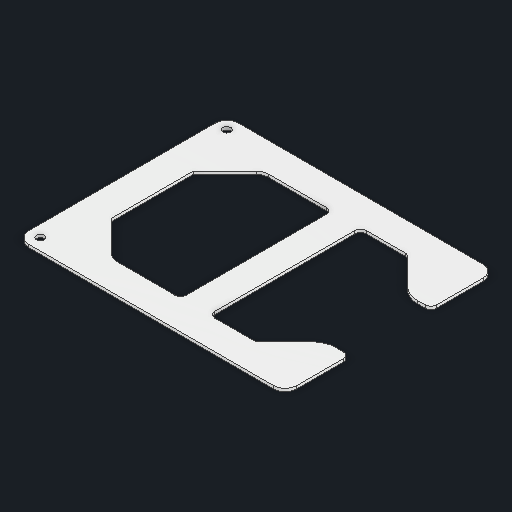
# Autodesk Inventor part: Compression Pads
Saved by Autodesk Inventor 2025.1 (Build 291241000, 241)
## iProperties
Created: 2024-11-12
Part Number: Compression Pads
Material: Acetal Resin, White
Document SubType Name: Sheet Metal
Designer: avere
Density: 1.425 g/cm^3
Appearance: Smooth - White
Flat Pattern Width: 11.43 cm
Flat Pattern Length: 14.605 cm
Flat Pattern Area: 166.935 cm^2
Sheet Metal Rule: Default_mm
Sheet Metal Width: 4.500 in
Sheet Metal Length: 5.750 in
Sheet Metal Area: 25.875 in^2
Author: avere
Autodesk Inventor part; units mm, degrees
ref_plane "YZ Plane" through (0, 0, 0) normal (1, 0, 0) x (0, 1, 0)
ref_plane "XZ Plane" through (0, 0, 0) normal (0, 1, 0) x (-1, 0, 0)
ref_plane "XY Plane" through (0, 0, 0) normal (0, 0, 1) x (1, 0, 0)
sketch "Sketch1" plane through (0, 0, 0) normal (0, 1, 0) x (-1, 0, 0)
  circle A0 centre (72.0639, -46.9126) radius 2.1844
  circle A1 centre (72.0639, 54.6874) radius 2.1844
  arc A2 (72.0639, -53.2626) -> (78.4139, -46.9126) centre (72.0639, -46.9126) ccw
  arc A3 (78.4139, 54.6874) -> (72.0639, 61.0374) centre (72.0639, 54.6874) ccw
  line L0 (78.4139, 54.6874) -> (78.4139, -46.9126)
  line L1 (72.0639, 61.0374) -> (-61.2861, 61.0374)
  line L2 (-67.6361, 54.6874) -> (-67.6361, 45.1624)
  line L3 (61.7451, 26.1124) -> (61.7451, -18.3376)
  line L4 (-67.6361, -37.3876) -> (-67.6361, -46.9126)
  line L5 (-61.2861, -53.2626) -> (72.0639, -53.2626)
  line L6 (55.3951, -37.3876) -> (61.7451, -31.0376)
  line L7 (44.555, -35.5277) -> (61.7451, -18.3376)
  line L8 (44.555, 43.3025) -> (61.7451, 26.1124)
  line L9 (-67.6361, -53.2626) -> (-67.6361, -21.5126)
  line L10 (-64.4611, -18.3376) -> (-60.1966, -18.3376)
  line L11 (-51.2164, -22.0573) -> (-36.8161, -36.4577)
  line L12 (-67.6361, 61.0374) -> (-67.6361, 29.2874)
  line L13 (-64.4611, 26.1124) -> (-60.1966, 26.1124)
  line L14 (-51.2164, 29.8321) -> (-36.8161, 44.2325)
  line L15 (-10.3147, 41.9874) -> (-10.3147, -34.2126)
  line L16 (5.0881, 41.9874) -> (5.0881, -34.2126)
  line L17 (40.0649, -37.3876) -> (8.2631, -37.3876)
  line L18 (-13.4897, -37.3876) -> (-34.571, -37.3876)
  line L19 (-34.571, 45.1624) -> (-13.4897, 45.1624)
  line L20 (8.2631, 45.1624) -> (40.0649, 45.1624)
  arc A4 (5.0881, -34.2126) -> (8.2631, -37.3876) centre (8.2631, -34.2126) ccw
  arc A5 (-13.4897, -37.3876) -> (-10.3147, -34.2126) centre (-13.4897, -34.2126) ccw
  arc A6 (-36.8161, -36.4577) -> (-34.571, -37.3876) centre (-34.571, -34.2126) ccw
  arc A7 (-51.2164, -22.0573) -> (-60.1966, -18.3376) centre (-60.1966, -31.0376) ccw
  arc A8 (-60.1966, 26.1124) -> (-51.2164, 29.8321) centre (-60.1966, 38.8124) ccw
  arc A9 (8.2631, 45.1624) -> (5.0881, 41.9874) centre (8.2631, 41.9874) ccw
  arc A10 (-10.3147, 41.9874) -> (-13.4897, 45.1624) centre (-13.4897, 41.9874) ccw
  arc A11 (-34.571, 45.1624) -> (-36.8161, 44.2325) centre (-34.571, 41.9874) ccw
  arc A12 (-67.6361, 29.2874) -> (-64.4611, 26.1124) centre (-64.4611, 29.2874) ccw
  arc A13 (-64.4611, -18.3376) -> (-67.6361, -21.5126) centre (-64.4611, -21.5126) ccw
  arc A14 (-67.6361, -46.9126) -> (-61.2861, -53.2626) centre (-61.2861, -46.9126) ccw
  arc A15 (-61.2861, 61.0374) -> (-67.6361, 54.6874) centre (-61.2861, 54.6874) ccw
  arc A16 (44.555, 43.3025) -> (40.0649, 45.1624) centre (40.0649, 38.8124) ccw
  arc A17 (40.0649, -37.3876) -> (44.555, -35.5277) centre (40.0649, -31.0376) ccw
  point P0 (0, 0)
  point P1 (61.7451, 45.1624)
  point P2 (61.7451, -37.3876)
  point P3 (42.6951, -37.3876)
  point P4 (61.7451, -37.3876)
  point P5 (42.6951, 45.1624)
  point P6 (-67.6361, -18.3376)
  point P7 (-54.9361, -18.3376)
  dimension "d0" = 4.3688
  dimension "d1" = 4.3688
  dimension "d2" = 12.7
  dimension "d3" = 12.7
  dimension "d4" = 139.7
  dimension "d5" = 6.35
  dimension "d6" = 6.35
  dimension "d7" = 19.05
  dimension "d8" = 19.05
  dimension "d9" = 19.05
  dimension "d10" = 19.05
  dimension "d11" = 12.7
  dimension "d12" = 135
  dimension "d13" = 3.175
  dimension "d14" = 12.7
  dimension "d15" = 6.35
  constraints: 42 end point, 32 point on circle, 31 tangent, 19 point on line, 18 centre point, 11 equal radius, 11 perpendicular, 2 coincident, 1 horizontal, 1 parallel, 1 vertical
  measures "d0" diameter of A0
  measures "d1" diameter of A1
  measures "d2" diameter of A2
  measures "d3" diameter of A3
  measures "d4" distance of L1.start L12.start
  measures "d5" distance of L6.start point (61.745, -37.388)
  measures "d6" distance of L6.end point (61.745, -37.388)
  measures "d7" distance of point (42.695, -37.388) point (61.745, -37.388)
  measures "d8" distance of L3.end point (61.745, -37.388)
  measures "d9" distance of point (42.695, 45.162) point (61.745, 45.162)
  measures "d10" distance of L8.end point (61.745, 45.162)
  measures "d11" distance of point (-67.636, -18.338) point (-54.936, -18.338)
  measures "d12" angle of L10 L11
  measures "d13" radius of A4
  measures "d14" radius of A7
  measures "d15" radius of A14
extrude "Extrusion1" add sketch "Sketch1" along normal blind 1.5875
feature "Bend Part1" [suppressed]
feature "Bend Part2" [suppressed]
equation "\"d6\" = d5"
equation "\"d8\" = d7"
equation "\"d9\" = d7"
equation "\"d10\" = d9"
equation "\"BendRadius\" = Thickness"
equation "\"BendReliefWidth\" = Thickness"
equation "\"BendReliefDepth\" = 0.5 * Thickness"
equation "\"CornerReliefSize\" = 4 * Thickness"
equation "\"MinimumRemnant\" = 2 * Thickness"
equation "\"TransitionRadius\" = BendRadius"
equation "\"JacobiRadiusSize\" = BendRadius"
equation "\"GapSize\" = Thickness"
equation "\"Thickness\" = 1.5875"
body "Solid1"
